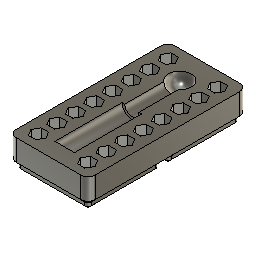
Gridfinity Hex Bit Holder 2x1 (Autodesk Fusion 360 design; units mm, degrees)
Autodesk Fusion 360 part; units mm, degrees
ref_plane "WorkPlane1" through (0, 0, 0) normal (0, 0, 1) x (1, 0, 0) in component "Gridfinity bin 2x1x2"
sketch "Sketch1" plane through (0, 0, 0) normal (0, 0, 1) x (1, 0, 0) in component "Gridfinity bin 2x1x2"
  line L0 (0, 0) -> (41.5, 0)
  line L1 (41.5, 0) -> (41.5, 41.5)
  line L2 (41.5, 41.5) -> (0, 41.5)
  line L3 (0, 41.5) -> (0, 0)
  dimension "d2" = 41.5
  dimension "d3" = 41.5
  constraint horizontal L0
  constraint vertical L1
  constraint horizontal L2
  constraint vertical L3
  constraint coincident L0.start L3
  constraint coincident L3.end L0
  measures "d2" horizontal distance of L0.start L0.end
  measures "d3" vertical distance of L0.end L1.end
extrude "Extrude1" add sketch "Sketch1" against normal blind 2.15 makes body 1 in component "Gridfinity bin 2x1x2"
fillet "Fillet1" radius 3.75 8 edges at (0, 0, -1.075) (41.5, 0, -1.075) (41.5, 0, -1.075) (41.5, 41.5, -1.075) (41.5, 41.5, -1.075) (0, 41.5, -1.075) (0, 41.5, -1.075) (0, 0, -1.075) on bodies 1 in component "Gridfinity bin 2x1x2"
chamfer "Chamfer1" distance 2.15 angle 45 8 edges at (1.0983, 40.4017, -2.15) (0, 20.75, -2.15) (1.0983, 1.0983, -2.15) (20.75, 0, -2.15) (40.4017, 1.0983, -2.15) (41.5, 20.75, -2.15) (40.4017, 40.4017, -2.15) (20.75, 41.5, -2.15) on bodies 1 in component "Gridfinity bin 2x1x2"
extrude "Extrude2" add 1 faces at (14.5499, 26.4167, -2.15) along direction (0, 0, -1) blind 2.6 on bodies 1 bodies 1 in component "Gridfinity bin 2x1x2"
chamfer "Chamfer2" distance 0.8 angle 45 8 edges at (2.6186, 38.8814, -4.75) (20.75, 39.35, -4.75) (38.8814, 38.8814, -4.75) (39.35, 20.75, -4.75) (38.8814, 2.6186, -4.75) (20.75, 2.15, -4.75) (2.6186, 2.6186, -4.75) (2.15, 20.75, -4.75) on bodies 1 in component "Gridfinity bin 2x1x2"
ref_plane "WorkPlane2" through (20.75, 20.75, -4.75) normal (0, 0, -1) x (-1, 0, 0) in component "Gridfinity bin 2x1x2"
sketch "Sketch2" plane through (20.75, 20.75, -4.75) normal (0, 0, -1) x (-1, 0, 0) in component "Gridfinity bin 2x1x2"
  circle A0 centre (13, -13) radius 3.25
  dimension "d13" = 6.5
  dimension "d14" = 13
  dimension "d15" = 13
  measures "d13" diameter of A0
  measures "d14" horizontal distance of origin A0.centre
  measures "d15" vertical distance of origin A0.centre
extrude "Extrude3" add sketch "Sketch2" against normal blind 2.4 separate body makes body 2 in component "Gridfinity bin 2x1x2"
pattern_linear "R-Pattern1" count 2 spacing 26 along (1, 0, 0) count 2 spacing 26 along (0, 1, 0) of bodies 2 makes body 3 at (30.5161, 7.4264, -3.95) makes body 4 at (4.5161, 33.4264, -3.95) makes body 5 at (30.5161, 33.4264, -3.95) in component "Gridfinity bin 2x1x2"
combine "Combine1" operation cut target body 1 tool bodies 2 3 4 5 2 in component "Gridfinity bin 2x1x2"
pattern_linear "R-Pattern2" count 1 spacing 42 along (1, 0, 0) count 2 spacing 42 along (0, 1, 0) of bodies 1 makes body 6 in component "Gridfinity bin 2x1x2"
sketch "Sketch3" plane through (0, 0, 0) normal (0, 0, 1) x (1, 0, 0) in component "Gridfinity bin 2x1x2"
  line L0 (0, 0) -> (41.5, 0)
  line L1 (41.5, 0) -> (41.5, 83.5)
  line L2 (41.5, 83.5) -> (0, 83.5)
  line L3 (0, 83.5) -> (0, 0)
  dimension "d26" = 41.5
  dimension "d27" = 83.5
  constraint horizontal L0
  constraint vertical L1
  constraint horizontal L2
  constraint vertical L3
  constraint coincident L0.start L3
  constraint coincident L3.end L0
  measures "d26" horizontal distance of L0.start L0.end
  measures "d27" vertical distance of L0.end L1.end
extrude "Extrude4" add sketch "Sketch3" along normal blind 11.21 separate body makes body 7 in component "Gridfinity bin 2x1x2"
fillet "Fillet2" radius 3.75 8 edges at (0, 83.5, 5.605) (41.5, 83.5, 5.605) (41.5, 83.5, 5.605) (41.5, 0, 5.605) (0, 0, 5.605) (0, 83.5, 5.605) (41.5, 0, 5.605) (0, 0, 5.605) on bodies 7 in component "Gridfinity bin 2x1x2"
combine "Combine2" operation add target body 7 tool bodies 1 6 1 in component "Gridfinity bin 2x1x2"
sketch "Sketch1 (2)" plane through (0, 0, 11.21) normal (0, 0, 1) x (-1, 0, 0)
  arc A0 (0, -3.75) -> (-3.75, 0) centre (-3.75, -3.75) ccw
  line L0 (-3.75, 0) -> (-37.75, 0)
  arc A1 (-37.75, 0) -> (-41.5, -3.75) centre (-37.75, -3.75) ccw
  line L1 (-41.5, -3.75) -> (-41.5, -79.75)
  arc A2 (-41.5, -79.75) -> (-37.75, -83.5) centre (-37.75, -79.75) ccw
  line L2 (-37.75, -83.5) -> (-3.75, -83.5)
  arc A3 (-3.75, -83.5) -> (0, -79.75) centre (-3.75, -79.75) ccw
  line L3 (0, -79.75) -> (0, -3.75)
  line L4 (-15.625, -8.5) -> (-25.875, -8.5)
  line L5 (-25.875, -8.5) -> (-25.875, -43.75)
  line L6 (-25.875, -43.75) -> (-15.625, -43.75)
  line L7 (-15.625, -43.75) -> (-15.625, -8.5)
  line L8 (-17.025, -43.75) -> (-24.475, -43.75)
  line L9 (-24.475, -43.75) -> (-24.475, -69)
  line L10 (-24.475, -69) -> (-17.025, -69)
  line L11 (-17.025, -69) -> (-17.025, -43.75)
  circle A4 centre (-20.75, -69) radius 6
  line L12 (-20.75, -8.5) -> (-20.75, 0) construction
  line L13 (-20.75, -75) -> (-20.75, -83.5) construction
  line L14 (-9.7611, -11) -> (-5.8639, -11)
  line L15 (-5.8639, -11) -> (-3.9154, -7.625)
  line L16 (-3.9154, -7.625) -> (-5.8639, -4.25)
  line L17 (-5.8639, -4.25) -> (-9.7611, -4.25)
  line L18 (-9.7611, -4.25) -> (-11.7096, -7.625)
  line L19 (-11.7096, -7.625) -> (-9.7611, -11)
  line L20 (-3.9154, -17.375) -> (-5.8639, -14)
  line L21 (-5.8639, -14) -> (-9.7611, -14)
  line L22 (-9.7611, -14) -> (-11.7096, -17.375)
  line L23 (-11.7096, -17.375) -> (-9.7611, -20.75)
  line L24 (-9.7611, -20.75) -> (-5.8639, -20.75)
  line L25 (-5.8639, -20.75) -> (-3.9154, -17.375)
  line L26 (-3.9154, -27.125) -> (-5.8639, -23.75)
  line L27 (-5.8639, -23.75) -> (-9.7611, -23.75)
  line L28 (-9.7611, -23.75) -> (-11.7096, -27.125)
  line L29 (-11.7096, -27.125) -> (-9.7611, -30.5)
  line L30 (-9.7611, -30.5) -> (-5.8639, -30.5)
  line L31 (-5.8639, -30.5) -> (-3.9154, -27.125)
  line L32 (-3.9154, -36.875) -> (-5.8639, -33.5)
  line L33 (-5.8639, -33.5) -> (-9.7611, -33.5)
  line L34 (-9.7611, -33.5) -> (-11.7096, -36.875)
  line L35 (-11.7096, -36.875) -> (-9.7611, -40.25)
  line L36 (-9.7611, -40.25) -> (-5.8639, -40.25)
  line L37 (-5.8639, -40.25) -> (-3.9154, -36.875)
  line L38 (-3.9154, -46.625) -> (-5.8639, -43.25)
  line L39 (-5.8639, -43.25) -> (-9.7611, -43.25)
  line L40 (-9.7611, -43.25) -> (-11.7096, -46.625)
  line L41 (-11.7096, -46.625) -> (-9.7611, -50)
  line L42 (-9.7611, -50) -> (-5.8639, -50)
  line L43 (-5.8639, -50) -> (-3.9154, -46.625)
  line L44 (-3.9154, -56.375) -> (-5.8639, -53)
  line L45 (-5.8639, -53) -> (-9.7611, -53)
  line L46 (-9.7611, -53) -> (-11.7096, -56.375)
  line L47 (-11.7096, -56.375) -> (-9.7611, -59.75)
  line L48 (-9.7611, -59.75) -> (-5.8639, -59.75)
  line L49 (-5.8639, -59.75) -> (-3.9154, -56.375)
  line L50 (-3.9154, -66.125) -> (-5.8639, -62.75)
  line L51 (-5.8639, -62.75) -> (-9.7611, -62.75)
  line L52 (-9.7611, -62.75) -> (-11.7096, -66.125)
  line L53 (-11.7096, -66.125) -> (-9.7611, -69.5)
  line L54 (-9.7611, -69.5) -> (-5.8639, -69.5)
  line L55 (-5.8639, -69.5) -> (-3.9154, -66.125)
  line L56 (-3.9154, -75.875) -> (-5.8639, -72.5)
  line L57 (-5.8639, -72.5) -> (-9.7611, -72.5)
  line L58 (-9.7611, -72.5) -> (-11.7096, -75.875)
  line L59 (-11.7096, -75.875) -> (-9.7611, -79.25)
  line L60 (-9.7611, -79.25) -> (-5.8639, -79.25)
  line L61 (-5.8639, -79.25) -> (-3.9154, -75.875)
  line L62 (-7.8125, -4.25) -> (-7.8125, 0) construction
  line L63 (-7.8125, -79.25) -> (-7.8125, -83.5) construction
  line L64 (-3.9154, -7.625) -> (0, -7.625) construction
  line L65 (-11.7096, -17.375) -> (-15.625, -17.375) construction
  line L66 (-35.6361, -4.25) -> (-31.7389, -4.25)
  line L67 (-31.7389, -4.25) -> (-29.7904, -7.625)
  line L68 (-29.7904, -7.625) -> (-31.7389, -11)
  line L69 (-31.7389, -11) -> (-35.6361, -11)
  line L70 (-37.5846, -7.625) -> (-35.6361, -4.25)
  line L71 (-35.6361, -11) -> (-37.5846, -7.625)
  line L72 (-31.7389, -14) -> (-29.7904, -17.375)
  line L73 (-29.7904, -17.375) -> (-31.7389, -20.75)
  line L74 (-31.7389, -20.75) -> (-35.6361, -20.75)
  line L75 (-35.6361, -20.75) -> (-37.5846, -17.375)
  line L76 (-35.6361, -14) -> (-31.7389, -14)
  line L77 (-37.5846, -17.375) -> (-35.6361, -14)
  line L78 (-31.7389, -23.75) -> (-29.7904, -27.125)
  line L79 (-29.7904, -27.125) -> (-31.7389, -30.5)
  line L80 (-31.7389, -30.5) -> (-35.6361, -30.5)
  line L81 (-35.6361, -30.5) -> (-37.5846, -27.125)
  line L82 (-35.6361, -23.75) -> (-31.7389, -23.75)
  line L83 (-37.5846, -27.125) -> (-35.6361, -23.75)
  line L84 (-31.7389, -33.5) -> (-29.7904, -36.875)
  line L85 (-29.7904, -36.875) -> (-31.7389, -40.25)
  line L86 (-31.7389, -40.25) -> (-35.6361, -40.25)
  line L87 (-35.6361, -40.25) -> (-37.5846, -36.875)
  line L88 (-35.6361, -33.5) -> (-31.7389, -33.5)
  line L89 (-37.5846, -36.875) -> (-35.6361, -33.5)
  line L90 (-31.7389, -43.25) -> (-29.7904, -46.625)
  line L91 (-29.7904, -46.625) -> (-31.7389, -50)
  line L92 (-31.7389, -50) -> (-35.6361, -50)
  line L93 (-35.6361, -50) -> (-37.5846, -46.625)
  line L94 (-35.6361, -43.25) -> (-31.7389, -43.25)
  line L95 (-37.5846, -46.625) -> (-35.6361, -43.25)
  line L96 (-31.7389, -53) -> (-29.7904, -56.375)
  line L97 (-29.7904, -56.375) -> (-31.7389, -59.75)
  line L98 (-31.7389, -59.75) -> (-35.6361, -59.75)
  line L99 (-35.6361, -59.75) -> (-37.5846, -56.375)
  line L100 (-35.6361, -53) -> (-31.7389, -53)
  line L101 (-37.5846, -56.375) -> (-35.6361, -53)
  line L102 (-31.7389, -62.75) -> (-29.7904, -66.125)
  line L103 (-29.7904, -66.125) -> (-31.7389, -69.5)
  line L104 (-31.7389, -69.5) -> (-35.6361, -69.5)
  line L105 (-35.6361, -69.5) -> (-37.5846, -66.125)
  line L106 (-35.6361, -62.75) -> (-31.7389, -62.75)
  line L107 (-37.5846, -66.125) -> (-35.6361, -62.75)
  line L108 (-31.7389, -72.5) -> (-29.7904, -75.875)
  line L109 (-29.7904, -75.875) -> (-31.7389, -79.25)
  line L110 (-31.7389, -79.25) -> (-35.6361, -79.25)
  line L111 (-35.6361, -79.25) -> (-37.5846, -75.875)
  line L112 (-35.6361, -72.5) -> (-31.7389, -72.5)
  line L113 (-37.5846, -75.875) -> (-35.6361, -72.5)
  point P0 (-7.8125, -7.625)
  dimension "d48" = 10.25
  dimension "d49" = 35.25
  dimension "d51" = 25.25
  dimension "d52" = 12
  dimension "d53" = 7.45
  dimension "d54" = 3.375
  dimension "d57" = 0
  dimension "d58" = -9.75
  constraint horizontal L4
  constraint vertical L5
  constraint horizontal L6
  constraint vertical L7
  constraint horizontal L8
  constraint vertical L9
  constraint horizontal L10
  constraint vertical L11
  constraint coincident L6 L8.start
  constraint midpoint L6 L8
  constraint midpoint L10 A4.centre
  constraint midpoint L4 L12.start
  constraint coincident L0 L12.end
  constraint perpendicular L0 L12
  constraint coincident A4 L13.start
  constraint midpoint L2 L13.end
  constraint perpendicular L2 L13
  constraint equal L12 L13
  constraint midpoint L0 L12.end
  constraint parallel L0 L17
  constraint midpoint L17 L62.start
  constraint coincident L0 L62.end
  constraint perpendicular L0 L62
  constraint coincident L2 L63.end
  constraint perpendicular L2 L63
  constraint equal L62 L63
  constraint coincident L3 L64.end
  constraint perpendicular L3 L64
  constraint coincident L7 L65.end
  constraint perpendicular L7 L65
  constraint equal L64 L65
  constraint coincident L60 L63.start
  constraint symmetric L12 L14.start L68.end
  constraint symmetric L12 L14.end L69.end
  constraint symmetric L12 L15.end L70.start
  constraint symmetric L12 L16.end L66.start
  constraint symmetric L12 L17.end L66.end
  constraint symmetric L12 L18.end L67.end
  constraint symmetric L12 L20.start L75.end
  constraint symmetric L12 L20.end L76.start
  constraint symmetric L12 L21.end L72.start
  constraint symmetric L12 L22.end L72.end
  constraint symmetric L12 L23.end L73.end
  constraint symmetric L12 L24.end L74.end
  constraint symmetric L12 L26.start L81.end
  constraint symmetric L12 L26.end L82.start
  constraint symmetric L12 L27.end L78.start
  constraint symmetric L12 L28.end L78.end
  constraint symmetric L12 L29.end L79.end
  constraint symmetric L12 L30.end L80.end
  constraint symmetric L12 L32.start L87.end
  constraint symmetric L12 L32.end L88.start
  constraint symmetric L12 L33.end L84.start
  constraint symmetric L12 L34.end L84.end
  constraint symmetric L12 L35.end L85.end
  constraint symmetric L12 L36.end L86.end
  constraint symmetric L12 L38.start L93.end
  constraint symmetric L12 L38.end L94.start
  constraint symmetric L12 L39.end L90.start
  constraint symmetric L12 L40.end L90.end
  constraint symmetric L12 L41.end L91.end
  constraint symmetric L12 L42.end L92.end
  constraint symmetric L12 L44.start L99.end
  constraint symmetric L12 L44.end L100.start
  constraint symmetric L12 L45.end L96.start
  constraint symmetric L12 L46.end L96.end
  constraint symmetric L12 L47.end L97.end
  constraint symmetric L12 L48.end L98.end
  constraint symmetric L12 L50.start L105.end
  constraint symmetric L12 L50.end L106.start
  constraint symmetric L12 L51.end L102.start
  constraint symmetric L12 L52.end L102.end
  constraint symmetric L12 L53.end L103.end
  constraint symmetric L12 L54.end L104.end
  constraint symmetric L12 L56.start L111.end
  constraint symmetric L12 L56.end L112.start
  constraint symmetric L12 L57.end L108.start
  constraint symmetric L12 L58.end L108.end
  constraint symmetric L12 L59.end L109.end
  constraint symmetric L12 L60.end L110.end
  measures "d48" distance of L4.start L4.end
  measures "d49" distance of L4.start L6.end
  measures "d51" distance of L8.start L10.end
  measures "d52" diameter of A4
  measures "d53" distance of L8.start L8.end
  measures "d54" distance of P0 L19
extrude "Extrude6" cut sketch "Sketch1 (2)" against normal blind 10 contours L14 L15 L16 L17 L18 L19 | L20 L21 L22 L23 L24 L25 | L26 L27 L28 L29 L30 L31 | L32 L33 L34 L35 L36 L37 | L38 L39 L40 L41 L42 L43 | L44 L45 L46 L47 L48 L49 | L50 L51 L52 L53 L54 L55 | L56 L57 L58 L59 L60 L61 | L66 L67 L68 L69 L70 L71 | L72 L73 L74 L75 L76 L77 | L78 L79 L80 L81 L82 L83 | L84 L85 L86 L87 L88 L89 | L90 L91 L92 L93 L94 L95 | L96 L97 L98 L99 L100 L101 | L102 L103 L104 L105 L106 L107 | L108 L109 L110 L111 L112 L113 bodies 7 in component "Gridfinity bin 2x1x2"
ref_plane "WorkPlane1" through (20.75, 8.5, 5.605) normal (0, -1, 0) x (1, 0, 0)
sketch "Sketch3 (2)" plane through (20.75, 8.5, 5.605) normal (0, -1, 0) x (1, 0, 0)
  circle A0 centre (0, 5.605) radius 5.125
  point P0 (0, 5.605)
  point P1 (-5.125, 5.605)
  constraint coincident P0 A0.centre
  constraint coincident A0 P1
extrude "Extrude7" cut sketch "Sketch3 (2)" against normal up to surface (35.25 mm away) bodies 7 in component "Gridfinity bin 2x1x2"
sketch "Sketch5" plane through (0, 43.75, 0) normal (0, -1, 0) x (1, 0, 0)
  line L0 (25.875, 11.21) -> (15.625, 11.21)
  arc A0 (15.625, 11.21) -> (25.875, 11.21) centre (20.75, 11.21) ccw
  circle A1 centre (20.75, 11.21) radius 3.725
  point P0 (17.025, 11.21)
  constraint concentric A0 A1
  constraint coincident A1 P0
extrude "Extrude8" cut sketch "Sketch5" against normal up to surface (25.25 mm away) contours L0 A1 | L0 A1 bodies 7 in component "Gridfinity bin 2x1x2"
sphere "SpherePrimitive1" cut diameter 12 placed x (-1, 0, 0) y (0, -1, 0) z (0, 0, 1) at (20.75, 69, 11.21) bodies 7 in component "Gridfinity bin 2x1x2"
component "Gridfinity bin 2x1x2" placed x (1, 0, 0) y (0, 1, 0) z (0, 0, 1) at (0, 0, 0)
equation "d4 = -( 2.15 mm )"
equation "WallOffset = 4 mm"
equation "d48 = 10 mm + Clearance"
equation "d49 = 35 mm + Clearance"
equation "Clearance = 0.25 mm"
equation "d51 = 25 mm + Clearance"
equation "d53 = 7.2 mm + Clearance"
equation "d54 = ( 6.25 / 2 ) * 1 mm + Clearance"
equation "d58 = -( 6.25 mm + 2 * Clearance ) - ( 0.5 * 6 ) * 1 mm"
named bodies: "base", "base (1)", "Gridfinity bin 2x1x2"
